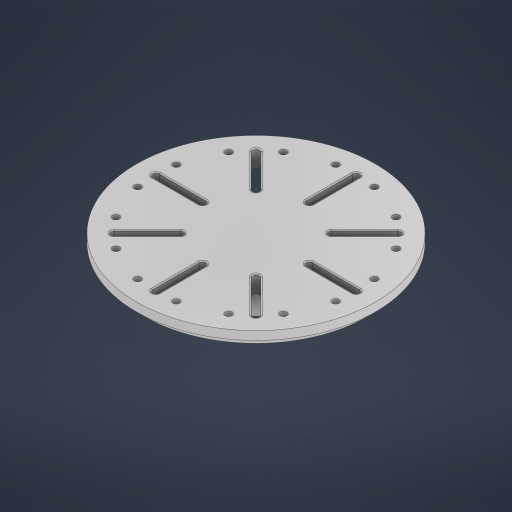
# Autodesk Inventor part: BaxisStol
Saved by Autodesk Inventor 2024 (Build 280153000, 153)
## iProperties
Created: 2023-12-23
Part Number: BaxisStol
Material: Aluminum 6061-AHC
Document SubType Name: Modeling
Designer: KirikDK
Mass: 12141 g
Surface Area: 3688.52 cm^2
Volume: 4496.67 cm^3
Density: 2.7 g/cm^3
Appearance: Aluminum - Dark
Author: KirikDK
Autodesk Inventor part; units mm, degrees
ref_plane "YZ Plane" through (0, 0, 0) normal (1, 0, 0) x (0, 1, 0)
ref_plane "XZ Plane" through (0, 0, 0) normal (0, 1, 0) x (-1, 0, 0)
ref_plane "XY Plane" through (0, 0, 0) normal (0, 0, 1) x (1, 0, 0)
sketch "Sketch1" plane through (0, 0, 0) normal (0, 1, 0) x (-1, 0, 0)
  circle A0 centre (0, 0) radius 80
  dimension "d0" = 160
  constraints: 1 centre point, 1 coincident
  measures "d0" diameter of A0
extrude "Extrusion1" add sketch "Sketch1" along normal blind 40
sketch "Sketch2" plane through (0, 40, 0) normal (0, 1, 0) x (1, 0, 0)
  circle A0 centre (0, 0) radius 210
  dimension "d3" = 420
  constraints: 1 centre point, 1 coincident
  measures "d3" diameter of A0
extrude "Extrusion2" add sketch "Sketch2" along normal blind 30
sketch "Sketch3" plane through (0, 70, 0) normal (0, 1, 0) x (1, 0, 0)
  line L0 (0, 94) -> (0, 176) construction
  line L1 (-6, 94) -> (-6, 176)
  line L2 (6, 176) -> (6, 94)
  arc A0 (-6, 94) -> (6, 94) centre (0, 94) ccw
  arc A1 (6, 176) -> (-6, 176) centre (0, 176) ccw
  circle A2 centre (34, 174) radius 6
  circle A3 centre (-34, 174) radius 6
  point P0 (0, 0)
  point P1 (0, 135)
  constraints: 8 end point, 4 centre point, 4 point on circle, 4 tangent, 1 midpoint, 1 parallel, 1 vertical
extrude "Extrusion3" cut sketch "Sketch3" against normal blind 30
pattern_circular "Circular Pattern1" count 8 over 360 about axis through (0, 40, 0) along (0, 1, 0) of "Extrusion3"
chamfer "Chamfer1" distance 15 angle 45 1 edges at (-210, 40, 0)
fillet "Fillet1" radius 2 32 edges at (-88, 70, 0) (-135, 70, 6) (-182, 70, 0) (-135, 70, -6) (-128.6934, 70, -128.6934) (-91.2168, 70, -99.7021) (-62.2254, 70, -62.2254) (-99.7021, 70, -91.2168) (0, 70, -182) (6, 70, -135) (0, 70, -88) (-6, 70, -135) (128.6934, 70, -128.6934) (99.7021, 70, -91.2168) (62.2254, 70, -62.2254) (91.2168, 70, -99.7021) (182, 70, 0) (135, 70, 6) (88, 70, 0) (135, 70, -6) (128.6934, 70, 128.6934) (91.2168, 70, 99.7021) (62.2254, 70, 62.2254) (99.7021, 70, 91.2168) (0, 70, 182) (-6, 70, 135) (0, 70, 88) (6, 70, 135) (-128.6934, 70, 128.6934) (-99.7021, 70, 91.2168) (-62.2254, 70, 62.2254) (-91.2168, 70, 99.7021)
body "Solid1"
